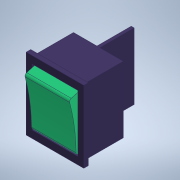
# Autodesk Inventor part: On_Off_Switch
Saved by Autodesk Inventor 2020 (Build 240168000, 168)
## iProperties
Created: 2019-06-07
Part Number: On_Off_Switch
Material: Generic
Document SubType Name: Modeling
Designer: LillaHunden
Density: 1 g/cm^3
Appearance: Default
Author: LillaHunden
Autodesk Inventor part; units mm, degrees
ref_plane "YZ Plane" through (0, 0, 0) normal (1, 0, 0) x (0, 1, 0)
ref_plane "XZ Plane" through (0, 0, 0) normal (0, 1, 0) x (-1, 0, 0)
ref_plane "XY Plane" through (0, 0, 0) normal (0, 0, 1) x (1, 0, 0)
sketch "Sketch1" plane through (0, 0, 0) normal (0, 0, 1) x (1, 0, 0)
  point P0 (0, 0)
sketch "Sketch2" plane through (0, 0, 0) normal (0, 0, 1) x (1, 0, 0)
  line L0 (-12.6, -15.7) -> (12.6, -15.7)
  line L1 (12.6, -15.7) -> (12.6, 15.7)
  line L2 (12.6, 15.7) -> (-12.6, 15.7)
  line L3 (-12.6, 15.7) -> (-12.6, -15.7)
  line L4 (-12.6, -15.7) -> (12.6, 15.7) construction
  line L5 (12.6, -15.7) -> (-12.6, 15.7) construction
  point P0 (0, 0)
  dimension "d0" = 25.2
  dimension "d1" = 31.4
  constraints: 12 end point, 2 midpoint, 2 parallel, 1 horizontal, 1 perpendicular
  measures "d0" distance of L2.end L1.end
  measures "d1" distance of L1.end L0.end
extrude "Extrusion1" add sketch "Sketch2" along normal blind 2
sketch "Sketch3" plane through (0, 0, 0) normal (0, 0, -1) x (-1, 0, 0)
  line L0 (-10.9, -14.5) -> (10.9, -14.5)
  line L1 (10.9, -14.5) -> (10.9, 14.5)
  line L2 (10.9, 14.5) -> (-10.9, 14.5)
  line L3 (-10.9, 14.5) -> (-10.9, -14.5)
  line L4 (-10.9, -14.5) -> (10.9, 14.5) construction
  line L5 (10.9, -14.5) -> (-10.9, 14.5) construction
  point P0 (0, 0)
  dimension "d4" = 21.8
  dimension "d5" = 29
  constraints: 12 end point, 2 midpoint, 2 parallel, 1 horizontal, 1 perpendicular
  measures "d4" distance of L2.end L1.end
  measures "d5" distance of L2.end L0.start
extrude "Extrusion2" add sketch "Sketch3" along normal blind 17
sketch "Sketch4" plane through (0, 0, -17) normal (0, 0, -1) x (-1, 0, 0)
  line L0 (-0.65, 14.5) -> (0.65, 14.5)
  line L1 (0.65, 14.5) -> (0.65, -14.5)
  line L2 (0.65, -14.5) -> (-0.65, -14.5)
  line L3 (-0.65, -14.5) -> (-0.65, 14.5)
  line L4 (-0.65, 14.5) -> (0.65, -14.5) construction
  line L5 (0.65, 14.5) -> (-0.65, -14.5) construction
  line L6 (-10.9, -14.5) -> (10.9, -14.5) projected
  point P0 (0, 0)
  point P1 (0, -14.5)
  dimension "d8" = 1.3
  constraints: 12 end point, 4 midpoint, 2 parallel, 1 horizontal, 1 perpendicular
  measures "d8" distance of L1.end L2.end
extrude "Extrusion3" add sketch "Sketch4" along normal blind 15
sketch "Sketch5" plane through (0, 0, 2) normal (0, 0, 1) x (1, 0, 0)
  line L0 (-10, -12.5) -> (10, -12.5)
  line L1 (10, -12.5) -> (10, 12.5)
  line L2 (10, 12.5) -> (-10, 12.5)
  line L3 (-10, 12.5) -> (-10, -12.5)
  line L4 (-10, -12.5) -> (10, 12.5) construction
  line L5 (10, -12.5) -> (-10, 12.5) construction
  point P0 (0, 0)
  dimension "d11" = 20
  dimension "d12" = 25
  constraints: 12 end point, 2 midpoint, 2 parallel, 1 horizontal, 1 perpendicular
  measures "d11" distance of L2.end L1.end
  measures "d12" distance of L1.end L0.end
extrude "Extrusion4" cut sketch "Sketch5" against normal blind 2
ref_plane "Work Plane1" through (0, -12.5, 2) normal (-1, 0, 0) x (0, 0, 1)
sketch "Sketch6" plane through (0, -12.5, 2) normal (-1, 0, 0) x (0, 0, 1)
  arc A0 (3.3287, 21.9761) -> (0.5045, 1.4881) centre (83.3994, 0.5) ccw
  line L0 (2.6334, 23.1979) -> (-2, 24.5)
  line L1 (-0.4954, 0.5) -> (-2, 0.5)
  line L2 (-2, 0) -> (-2, 25) projected
  arc A1 (3.3287, 21.9761) -> (2.6334, 23.1979) centre (2.3628, 22.2352) ccw
  arc A2 (-0.4954, 0.5) -> (0.5045, 1.4881) centre (-0.4954, 1.5) ccw
  line L3 (-2, 0.5) -> (-2, 24.5)
  point P0 (-2, 12.5)
  point P1 (3.5903, 22.9289)
  point P2 (0.4986, 0.5)
  dimension "d15" = 0.5
  dimension "d16" = 0.5
  dimension "d17" = 2.4986
  dimension "d18" = 5.5903
  dimension "d19" = 1
  constraints: 8 point on circle, 6 end point, 4 point on line, 4 tangent, 3 centre point, 2 line through centre, 1 collinear, 1 equal radius, 1 horizontal
  measures "d15" distance of L2.end L0.end
  measures "d16" distance of L2.start L1.end
  measures "d17" distance of point (0.499, 0.5) L1.end
  measures "d18" horizontal distance of point (3.59, 22.929) L0.end
  measures "d19" radius of A1
extrude "Extrusion5" add sketch "Sketch6" along normal mid plane 19.5
body "Solid1"
